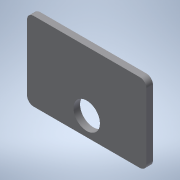
# Autodesk Inventor part: Standard
Saved by Autodesk Inventor 2020.3 (Build 243373000, 373)
## iProperties
RuleStatus: InUse
AfterDocSave0: file://Part Number Cleaner
Created: 2023-03-06
Material: Generic
Catalog Web Link: https://www.janelia.org/
Vendor: HHMI: JRC - jET
Document SubType Name: Modeling
Designer: jalala
Density: 1 g/cm^3
Appearance: Default
DESIGN DEPARTMENT: HHMI: JRC - jET
ALTERED ITEM PART NUMBER: N/A
ALTERED ITEM VENDOR: N/A
ALTERED ITEM DESCRIPTION: N/A
Title: Standard
Author: jalala
Revision Number: 0
Autodesk Inventor part; units mm, degrees
ref_plane "YZ Plane" through (0, 0, 0) normal (1, 0, 0) x (0, 1, 0)
ref_plane "XZ Plane" through (0, 0, 0) normal (0, 1, 0) x (-1, 0, 0)
ref_plane "XY Plane" through (0, 0, 0) normal (0, 0, 1) x (1, 0, 0)
sketch "Sketch1" plane through (0, 0, 0) normal (0, 0, 1) x (1, 0, 0)
  line L0 (-28.956, 18.0022) -> (-28.956, -40.1638) construction
  line L1 (28.956, 18.0022) -> (-28.956, 18.0022) construction
  line L2 (28.956, -40.1637) -> (28.956, 18.0022) construction
  line L3 (-25.781, 18.0022) -> (25.781, 18.0022)
  line L4 (28.956, 14.8272) -> (28.956, -16.9227)
  line L5 (25.781, -20.0977) -> (-25.781, -20.0978)
  line L6 (-28.956, -16.9228) -> (-28.956, 14.8272)
  arc A0 (-25.781, 18.0022) -> (-28.956, 14.8272) centre (-25.781, 14.8272) ccw
  arc A1 (28.956, 14.8272) -> (25.781, 18.0022) centre (25.781, 14.8272) ccw
  arc A2 (-28.956, -16.9228) -> (-25.781, -20.0978) centre (-25.781, -16.9228) ccw
  arc A3 (25.781, -20.0977) -> (28.956, -16.9227) centre (25.781, -16.9228) ccw
  circle A4 centre (0, -11.0808) radius 6.4135
  line L7 (-28.956, 18.0022) -> (28.956, -40.1637) construction
  line L8 (28.956, 18.0022) -> (-28.956, -40.1638) construction
  point P0 (0, 0)
  point P1 (28.956, -20.0977)
  point P2 (0, -11.0808)
  dimension "d0" = 38.1
  dimension "d1" = 3.175
  dimension "d2" = 12.827
  constraints: 12 end point, 8 point on circle, 8 tangent, 5 centre point, 5 point on line, 3 equal radius, 2 parallel, 1 coincident, 1 horizontal, 1 midpoint, 1 perpendicular
  measures "d0" distance between parallel lines of L1 L5
  measures "d1" radius of A0
  measures "d2" diameter of A4
extrude "Extrusion1" add sketch "Sketch1" against normal blind 3.175
body "Solid1"
